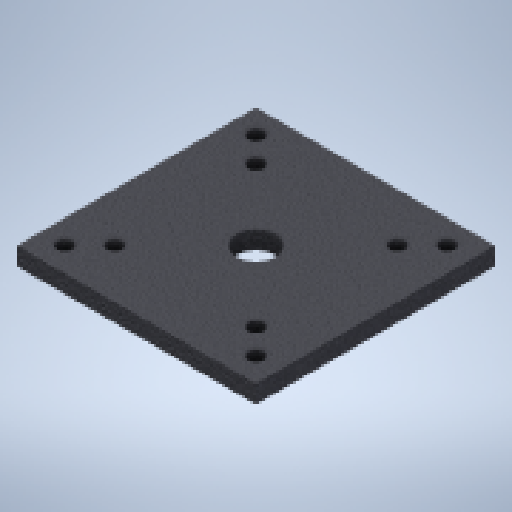
# Autodesk Inventor part: Suporte 1
Saved by Autodesk Inventor 2023 (Build 270158000, 158)
## iProperties
Created: 2023-03-21
Part Number: Suporte 1
Material: Aço
Document SubType Name: Sheet Metal
Designer: Mateus
Density: 7.85 g/cm^3
Sheet Metal Rule: Padrão_mm
Appearance: Ferro - Fundido
Author: Mateus
Autodesk Inventor part; units mm, degrees
ref_plane "YZ Plane" through (0, 0, 0) normal (1, 0, 0) x (0, 1, 0)
ref_plane "XZ Plane" through (0, 0, 0) normal (0, 1, 0) x (-1, 0, 0)
ref_plane "XY Plane" through (0, 0, 0) normal (0, 0, 1) x (1, 0, 0)
sketch "Esboço1" plane through (0, 0, 0) normal (0, 1, 0) x (-1, 0, 0)
  line L0 (0, 0) -> (80, 0)
  line L1 (80, 0) -> (80, -80)
  line L2 (80, -80) -> (0, -80)
  line L3 (0, -80) -> (0, 0)
  dimension "d0" = 80
  dimension "d1" = 80
  constraints: 8 end point, 2 parallel, 1 horizontal, 1 perpendicular
  measures "d0" distance of L1.end L2.end
  measures "d1" distance of L0.end L1.end
extrude "Extrusão1" add sketch "Esboço1" along normal blind 6
sketch "Esboço2" plane through (0, 6, 0) normal (0, 1, 0) x (1, 0, 0)
  line L0 (-80, 0) -> (0, 0) projected
  line L1 (0, 0) -> (0, 80) projected
  point P0 (-16.4, 16.4)
  point P1 (-16.4, 63.6)
  point P2 (-63.6, 63.6)
  point P3 (-63.6, 16.4)
  dimension "d4" = 47.2
  dimension "d5" = 47.2
  dimension "d6" = 47.2
  dimension "d7" = 47.2
  dimension "d8" = 0
  dimension "d9" = 0
  dimension "d10" = 80
  dimension "d11" = 16.4
  dimension "d12" = 16.4
  measures "d4" distance of point (-63.6, 16.4) point (-63.6, 63.6)
  measures "d5" distance of point (-16.4, 16.4) point (-63.6, 16.4)
  measures "d6" distance of point (-16.4, 63.6) point (-16.4, 16.4)
  measures "d7" distance of point (-16.4, 63.6) point (-63.6, 63.6)
  measures "d8" horizontal distance of point (-16.4, 16.4) point (-16.4, 63.6)
  measures "d9" vertical distance of point (-16.4, 16.4) point (-63.6, 16.4)
  measures "d10" distance of L0.start L0.end
  measures "d11" distance from line of L0 point (-16.4, 16.4)
  measures "d12" distance from line of L1 point (-16.4, 16.4)
hole "Furo1" at (-16.4, 6, -16.4) at (-16.4, 6, -63.6) at (-63.6, 6, -63.6) at (-63.6, 6, -16.4) direction (0, -1, 0) diameter 5 depth 6 tip angle 118
sketch "Esboço3" plane through (0, 6, 0) normal (0, 1, 0) x (1, 0, 0)
  line L0 (-80, 0) -> (0, 0) projected
  line L1 (-80, 80) -> (-80, 0) projected
  line L2 (0, 0) -> (0, 80) projected
  line L3 (0, 80) -> (-80, 80) projected
  point P0 (-8, 8)
  point P1 (-8, 72)
  point P2 (-72, 72)
  point P3 (-72, 8)
  dimension "d20" = 8
  dimension "d21" = 8
  dimension "d22" = 8
  dimension "d23" = 8
  dimension "d24" = 8
  dimension "d25" = 8
  dimension "d26" = 8
  dimension "d27" = 8
  measures "d20" distance from line of L0 point (-72, 8)
  measures "d21" distance from line of L1 point (-72, 8)
  measures "d22" distance from line of L1 point (-72, 72)
  measures "d23" distance from line of L2 point (-8, 8)
  measures "d24" distance from line of L0 point (-8, 8)
  measures "d25" distance from line of L3 point (-72, 72)
  measures "d26" distance from line of L3 point (-8, 72)
  measures "d27" distance from line of L2 point (-8, 72)
hole "Furo2" at (-8, 6, -8) at (-8, 6, -72) at (-72, 6, -72) at (-72, 6, -8) direction (0, -1, 0) diameter 5 depth 6 tip angle 118
sketch "Esboço4" plane through (0, 6, 0) normal (0, 1, 0) x (1, 0, 0)
  line L0 (-80, 80) -> (-80, 0) projected
  line L1 (-80, 0) -> (0, 0) projected
  point P0 (-40, 40)
  dimension "d35" = 80
  dimension "d36" = 40
  dimension "d37" = 40
  measures "d35" distance of L0.start L0.end
  measures "d36" distance from line of L0 point (-40, 40)
  measures "d37" distance from line of L1 point (-40, 40)
hole "Furo3" at (-40, 6, -40) direction (0, -1, 0) diameter 13 depth 6 tip angle 118
equation "\"d11\" = -0.5 * d4 + 0.5 * d10"
equation "\"d12\" = d11"
equation "\"d18\" = Espessura"
equation "\"d22\" = d21"
equation "\"d23\" = d20"
equation "\"d24\" = d21"
equation "\"d25\" = d20"
equation "\"d26\" = d25"
equation "\"d27\" = d23"
equation "\"d36\" = 0.5 * d35"
equation "\"d37\" = d36"
equation "\"Raio_vergadura\" = Espessura"
equation "\"Largura_alívio_de_vergadura\" = Espessura"
equation "\"Profundidade_alívio_de_vergadura\" = 0.5 * Espessura"
equation "\"Tamanho_alívio_de_dobra\" = 4 * Espessura"
equation "\"Remanescente_mínimo\" = 2 * Espessura"
equation "\"Raiodetransição\" = Raio_vergadura"
equation "\"Tamanho_de_raio_de_Jacobi\" = Raio_vergadura"
equation "\"TamanhoFolga\" = Espessura"
equation "\"Espessura\" = 0.5"
